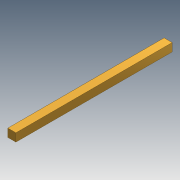
# Autodesk Inventor part: Straight Header Pin
Saved by Autodesk Inventor 2016 (Build 200138000, 138)
## iProperties
Created: 2016-01-25
Part Number: Straight Header Pin
Material: Brass, Soft Yellow
Document SubType Name: Modeling
Designer: larraguetajunior
Mass: 0.0353707 g
Surface Area: 0.2856 cm^2
Volume: 0.004176 cm^3
Density: 8.47 g/cm^3
Appearance: Brass - Satin
Author: larraguetajunior
Autodesk Inventor part; units mm, degrees
ref_plane "YZ Plane" through (0, 0, 0) normal (1, 0, 0) x (0, 1, 0)
ref_plane "XZ Plane" through (0, 0, 0) normal (0, 1, 0) x (-1, 0, 0)
ref_plane "XY Plane" through (0, 0, 0) normal (0, 0, 1) x (1, 0, 0)
sketch "Sketch1" plane through (0, 0, 0) normal (0, 1, 0) x (-1, 0, 0)
  line L0 (0.3, 0.3) -> (-0.3, 0.3)
  line L1 (-0.3, 0.3) -> (-0.3, -0.3)
  line L2 (-0.3, -0.3) -> (0.3, -0.3)
  line L3 (0.3, -0.3) -> (0.3, 0.3)
  line L4 (0.3, 0.3) -> (-0.3, -0.3) construction
  line L5 (-0.3, 0.3) -> (0.3, -0.3) construction
  point P0 (0, 0)
  dimension "d0" = 0.6
  dimension "d1" = 0.6
  constraints: 12 end point, 2 midpoint, 2 parallel, 1 horizontal, 1 perpendicular
  measures "d0" distance of L2.end L1.end
  measures "d1" distance of L1.end L0.end
extrude "Extrusion1" add sketch "Sketch1" along normal mid plane 11.6
body "Solid1"
